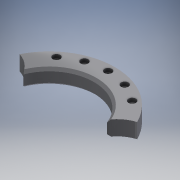
# Autodesk Inventor part: Funnel_Adapter
Saved by Autodesk Inventor 2016 (Build 200138000, 138)
## iProperties
Created: 2015-07-20
Part Number: Funnel_Adapter
Material: Generic
Document SubType Name: Modeling
Designer: bastli
Density: 1 g/cm^3
Appearance: Default
Author: bastli
Autodesk Inventor part; units mm, degrees
ref_plane "YZ Plane" through (0, 0, 0) normal (1, 0, 0) x (0, 1, 0)
ref_plane "XZ Plane" through (0, 0, 0) normal (0, 1, 0) x (-1, 0, 0)
ref_plane "XY Plane" through (0, 0, 0) normal (0, 0, 1) x (1, 0, 0)
derived "Transmission.ipt"
sketch "Sketch1" plane through (0, 0, 0) normal (0, 0, 1) x (1, 0, 0)
  circle A0 centre (-41.0929, -23.725) radius 1.55 construction
  circle A1 centre (-30.5003, -36.3488) radius 1.55 construction
  circle A2 centre (-21.1266, -58.0448) radius 1.55 construction
  circle A3 centre (0, -47.45) radius 1.55 construction
  circle A4 centre (16.2289, -44.5884) radius 1.55 construction
  circle A5 centre (39.705, -47.3186) radius 1.55 construction
  circle A6 centre (41.0929, -23.725) radius 1.55 construction
  circle A7 centre (-41.0929, 23.725) radius 1.55 construction
  circle A8 centre (-30.5003, 36.3488) radius 1.55 construction
  circle A9 centre (-16.2289, 44.5884) radius 1.55 construction
  circle A10 centre (53.4944, 30.885) radius 1.55 construction
  circle A11 centre (39.705, 47.3186) radius 1.55 construction
  circle A12 centre (21.1266, 58.0448) radius 1.55 construction
  circle A13 centre (0, 61.77) radius 1.55 construction
  circle A14 centre (0, 47.45) radius 1.55 construction
  circle A15 centre (16.2289, 44.5884) radius 1.55 construction
  circle A16 centre (30.5003, 36.3488) radius 1.55 construction
  circle A17 centre (41.0929, 23.725) radius 1.55 construction
  circle A18 centre (-21.1266, 58.0448) radius 1.55 construction
  circle A19 centre (-39.705, 47.3186) radius 1.55 construction
  circle A20 centre (-53.4944, 30.885) radius 1.55 construction
  circle A21 centre (53.4944, -30.885) radius 1.55 construction
  circle A22 centre (30.5003, -36.3488) radius 1.55 construction
  circle A23 centre (21.1266, -58.0448) radius 1.55 construction
  circle A24 centre (0, -61.77) radius 1.55 construction
  circle A25 centre (-16.2289, -44.5884) radius 1.55 construction
  circle A26 centre (-39.705, -47.3186) radius 1.55 construction
  circle A27 centre (-53.4944, -30.885) radius 1.55 construction
  circle A28 centre (62.61, 8) radius 3 construction
  circle A29 centre (46.61, -8) radius 3 construction
  circle A30 centre (-46.61, -8) radius 3 construction
  circle A31 centre (-62.61, 8) radius 3 construction
  circle A32 centre (-46.61, 8) radius 3 construction
  circle A33 centre (-62.61, -8) radius 3 construction
  circle A34 centre (46.61, 8) radius 3 construction
  circle A35 centre (62.61, -8) radius 3 construction
  circle A36 centre (-54.61, 0) radius 7.995 construction
  circle A37 centre (54.61, 0) radius 7.995 construction
  circle A38 centre (0, 0) radius 37.95 construction
  circle A39 centre (0, 0) radius 67.77 construction
  circle A40 centre (0, 0) radius 36 construction
  circle A41 centre (-54.61, 0) radius 21.61 construction
  circle A42 centre (54.61, 0) radius 21.61 construction
  circle A43 centre (-54.61, 0) radius 24.61 construction
  circle A44 centre (54.61, 0) radius 24.61 construction
  circle A45 centre (0, 0) radius 52.86 construction
  line L0 (0, 37.95) -> (0, 52.86) construction
  line L1 (0, 52.86) -> (0, 67.77) construction
  line L2 (0, 0) -> (0, 37.95) construction
  arc A46 (33.6257, 12.8574) -> (-33.6257, 12.8574) centre (0, 0) ccw
  circle A47 centre (54.61, 0) radius 2.1 projected
  arc A48 (47.3428, 23.5125) -> (33.6257, 12.8574) centre (54.61, 0) ccw
  arc A49 (47.3428, 23.5125) -> (-47.3428, 23.5125) centre (0, 0) ccw
  arc A50 (-33.6257, 12.8574) -> (-47.3428, 23.5125) centre (-54.61, 0) ccw
  point P0 (0, 0)
  dimension "d0" = 72
  dimension "d3" = 43.22
  dimension "d4" = 43.22
  dimension "d6" = 3
  dimension "d7" = 3
  constraints: 20 coincident, 10 point on circle, 7 centre point, 6 end point, 2 vertical, 2 vertical alignment, 1 collinear, 1 point on line, 11 other
  measures "d3" diameter of A41
  measures "d4" diameter of A42
extrude "Extrusion1" add sketch "Sketch1" along normal blind 12.7 contours A46 A50 A49 A48
sketch "Sketch2" plane through (0, 0, 12.7) normal (0, 0, 1) x (1, 0, 0)
  circle A0 centre (-30.5003, 36.3488) radius 1.55 projected
  circle A1 centre (-16.2289, 44.5884) radius 1.55 projected
  circle A2 centre (0, 47.45) radius 1.55 projected
  circle A3 centre (16.2289, 44.5884) radius 1.55 projected
  circle A4 centre (30.5003, 36.3488) radius 1.55 projected
  point P0 (0, 0)
  constraints: 5 coincident
hole "Hole1" at (-30.5003, 36.3488, 12.7) at (0, 47.45, 12.7) at (30.5003, 36.3488, 12.7) at (16.2289, 44.5884, 12.7) at (-16.2289, 44.5884, 12.7) direction (0, 0, -1) diameter 3.1 end through all
hole "Hole2" at (-30.5003, 36.3488, 12.7) at (-16.2289, 44.5884, 12.7) at (0, 47.45, 12.7) at (16.2289, 44.5884, 12.7) at (30.5003, 36.3488, 12.7) direction (0, 0, -1) diameter 6 depth 3
chamfer "Chamfer1" distance 2 angle 45 1 edges at (0, 36, 0)
chamfer "Chamfer2" distance 2 angle 45 1 edges at (0, 36, 12.7)
equation "\"d0\" = funnel_width"
equation "\"d3\" = d5"
equation "\"d4\" = d5"
equation "\"d7\" = thickness"
equation "\"funnel_width\" = 72"
equation "\"thickness\" = 3"
equation "\"d5\" = 43.22"
body "Solid1"
